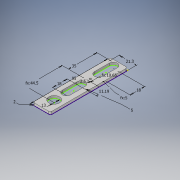
# Autodesk Inventor part: 12mero
Saved by Autodesk Inventor 2019 (Build 230136000, 136)
## iProperties
Created: 2022-09-04
Part Number: 12mero
Material: Generic
Document SubType Name: Modeling
Designer: laca
Density: 1 g/cm^3
Appearance: Default
Author: laca
Autodesk Inventor part; units mm, degrees
ref_plane "YZ Plane" through (0, 0, 0) normal (1, 0, 0) x (0, 1, 0)
ref_plane "XZ Plane" through (0, 0, 0) normal (0, 1, 0) x (-1, 0, 0)
ref_plane "XY Plane" through (0, 0, 0) normal (0, 0, 1) x (1, 0, 0)
sketch "Sketch1" plane through (0, 0, 0) normal (0, 1, 0) x (-1, 0, 0)
  line L0 (2, 0) -> (19.3, 0)
  line L1 (21.3, 2) -> (21.3, 93)
  line L2 (19.3, 95) -> (2, 95)
  line L3 (0, 93) -> (0, 2)
  circle A0 centre (10.65, 35) radius 1.25
  arc A1 (21.3, 93) -> (19.3, 95) centre (19.3, 93) ccw
  arc A2 (2, 95) -> (0, 93) centre (2, 93) ccw
  arc A3 (0, 2) -> (2, 0) centre (2, 2) ccw
  arc A4 (19.3, 0) -> (21.3, 2) centre (19.3, 2) ccw
  circle A5 centre (10.65, 79.5) radius 6.5
  line L4 (11, 46.1899) -> (11, 64.1899) construction
  line L5 (6, 46.1899) -> (6, 64.1899)
  line L6 (16, 64.1899) -> (16, 46.1899)
  arc A6 (6, 46.1899) -> (16, 46.1899) centre (11, 46.1899) ccw
  arc A7 (16, 64.1899) -> (6, 64.1899) centre (11, 64.1899) ccw
  line L7 (11, 6.6463) -> (11, 24.6463) construction
  line L8 (6, 6.6463) -> (6, 24.6463)
  line L9 (16, 24.6463) -> (16, 6.6463)
  arc A8 (6, 6.6463) -> (16, 6.6463) centre (11, 6.6463) ccw
  arc A9 (16, 24.6463) -> (6, 24.6463) centre (11, 24.6463) ccw
  point P0 (0, 0)
  point P1 (21.3, 95)
  point P2 (21.3, 0)
  point P3 (11, 55.1899)
  point P4 (11, 15.6463)
  dimension "d0" = 21.3
  dimension "d1" = 95
  dimension "d2" = 2.5
  dimension "d3" = 35
  dimension "d6" = 10.65
  dimension "d8" = 2
  dimension "d9" = 13
  dimension "d10" = 44.5
  dimension "d13" = 18
  dimension "d14" = 5
  dimension "d17" = 11.1898
  dimension "d18" = 18
  dimension "d19" = 5
  constraints: 24 end point, 16 point on circle, 16 tangent, 10 centre point, 6 point on line, 4 parallel, 3 equal radius, 2 midpoint, 2 vertical, 1 horizontal, 1 perpendicular
  measures "d0" distance between parallel lines of L3 L1
  measures "d1" distance of point (21.3, 0) point (21.3, 95)
  measures "d2" diameter of A0
  measures "d3" distance from line of L0 A0.centre
  measures "d6" distance from line of L3 A0.centre
  measures "d8" radius of A1
  measures "d9" diameter of A5
  measures "d10" distance of A0.centre A5.centre
  measures "d13" distance of L4.end L4.start
  measures "d14" radius of A6
  measures "d17" vertical distance of A0.centre L4.start
  measures "d18" distance of L7.end L7.start
  measures "d19" radius of A9
extrude "Extrusion1" add sketch "Sketch1" along normal blind 3 contours A3 L3 A2 L2 A1 L1 A4 L0 | L5 A7 L6 A6 | L8 A9 L9 A8
extrude "Extrusion2" cut sketch "Sketch1" along normal through all contours L5 A7 L6 A6 | L8 A9 L9 A8
equation "\"d6\" = 0.5 * d0"
equation "\"d19\" = d14"
body "Solid1"
